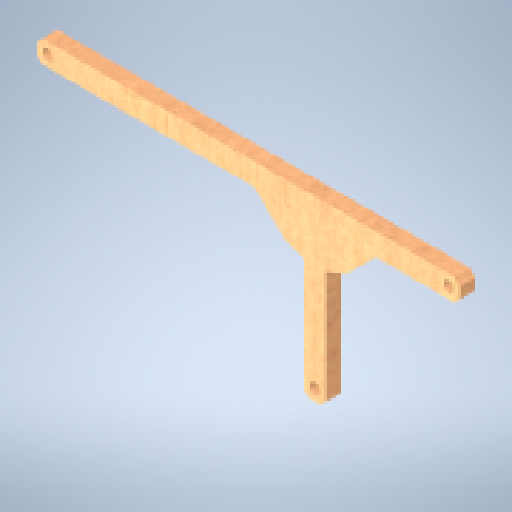
# Autodesk Inventor part: brazoT
Saved by Autodesk Inventor 2023.1 (Build 271208000, 208)
## iProperties
Created: 2022-10-30
Part Number: brazoT
Material: MDF Medium Density Fiberboard
Document SubType Name: Modeling
Designer: Daniel Peña
Density: 0.8 g/cm^3
Appearance: Cherry - Natural Low Gloss
Author: Daniel Peña
Autodesk Inventor part; units mm, degrees
ref_plane "YZ Plane" through (0, 0, 0) normal (1, 0, 0) x (0, 1, 0)
ref_plane "XZ Plane" through (0, 0, 0) normal (0, 1, 0) x (-1, 0, 0)
ref_plane "XY Plane" through (0, 0, 0) normal (0, 0, 1) x (1, 0, 0)
sketch "Sketch1" plane through (0, 0, 0) normal (0, 0, 1) x (1, 0, 0)
  circle A0 centre (-125, 70) radius 2.5 projected
  circle A1 centre (-185, 0.0856) radius 2.5 projected
  line L0 (-125, 70) -> (-305, 70) construction
  line L1 (-185, 0.0856) -> (-185, 70) construction
  line L2 (-310, 67.5) -> (-310, 72.5)
  line L3 (-307.5, 75) -> (-122.5, 75)
  line L4 (-120, 72.5) -> (-120, 67.5)
  line L5 (-180, 48.0357) -> (-180, -2.4144)
  line L6 (-182.5, -4.9144) -> (-187.5, -4.9144)
  line L7 (-190, -2.4144) -> (-190, 48.0357)
  line L8 (-122.5, 65) -> (-157.6881, 65)
  line L9 (-212.3119, 65) -> (-307.5, 65)
  line L10 (-120, 67.5) -> (-122.5, 65)
  line L11 (-120, 72.5) -> (-122.5, 75)
  line L12 (-180, -2.4144) -> (-182.5, -4.9144)
  line L13 (-187.5, -4.9144) -> (-190, -2.4144)
  line L14 (-307.5, 65) -> (-310, 67.5)
  line L15 (-307.5, 75) -> (-310, 72.5)
  line L16 (-170.7801, 51.9079) -> (-180, 48.0357)
  line L17 (-170.7801, 51.9079) -> (-157.6881, 65)
  line L18 (-199.2199, 51.9079) -> (-190, 48.0357)
  line L19 (-199.2199, 51.9079) -> (-212.3119, 65)
  point P0 (0, 0)
  point P1 (-120, 65)
  point P2 (-310, 75)
  point P3 (-310, 65)
  point P4 (-120, 75)
  point P5 (-180, -4.9144)
  point P6 (-190, -4.9144)
  point P7 (-161.5602, 55.7801)
  dimension "d0" = 180
  dimension "d1" = 60
  dimension "d2" = 5
  dimension "d3" = 5
  dimension "d4" = 5
  dimension "d5" = 5
  dimension "d6" = 5
  dimension "d7" = 2.5
  dimension "d8" = 2.5
  dimension "d9" = 2.5
  dimension "d10" = 2.5
  dimension "d11" = 2.5
  dimension "d12" = 2.5
  dimension "d13" = 2.5
  dimension "d14" = 2.5
  dimension "d15" = 2.5
  dimension "d16" = 2.5
  dimension "d17" = 2.5
  dimension "d18" = 2.5
  dimension "d19" = 20
  dimension "d20" = 10
  dimension "d21" = 10
  dimension "d22" = 10
  constraints: 40 end point, 14 point on line, 4 horizontal, 4 parallel, 3 perpendicular, 3 symmetric about line, 1 coincident, 1 collinear, 5 other
  measures "d0" distance of L0.start L0.end
  measures "d1" distance from line of L0.start L1
  measures "d2" distance between parallel lines of L3 L0
  measures "d3" distance from line of L0.start L4
  measures "d4" distance from line of L0.end L2
  measures "d5" distance between parallel lines of L5 L1
  measures "d6" distance from line of L1.start L6
  measures "d7" distance of L4.end point (-120, 65)
  measures "d8" distance of L8.start point (-120, 65)
  measures "d9" distance of L4.start point (-120, 75)
  measures "d10" distance of L3.end point (-120, 75)
  measures "d11" distance of L5.end point (-180, -4.914)
  measures "d12" distance of L6.start point (-180, -4.914)
  measures "d13" distance of L6.end point (-190, -4.914)
  measures "d14" distance of L7.start point (-190, -4.914)
  measures "d15" distance of L9.end point (-310, 65)
  measures "d16" distance of L2.start point (-310, 65)
  measures "d17" distance of L3.start point (-310, 75)
  measures "d18" distance of L2.end point (-310, 75)
  measures "d19" distance of L5.start point (-161.56, 55.78)
  measures "d20" distance of point (-157.688, 65) point (-161.56, 55.78)
  measures "d21" distance of L16.start point (-161.56, 55.78)
  measures "d22" distance of L8.end point (-161.56, 55.78)
extrude "Extrusion1" add sketch "Sketch1" along normal blind 7 contours A0 | A1 | L2 L15 L3 L11 L4 L10 L8 L17 L16 L5 L12 L6 L13 L7 L18 L19 L9 L14
sketch "Sketch2" plane through (0, 0, 7) normal (0, 0, 1) x (1, 0, 0)
  line L0 (-120, 67.5) -> (-120, 72.5) projected
  line L1 (-187.5, -4.9144) -> (-182.5, -4.9144) projected
  line L2 (-310, 72.5) -> (-310, 67.5) projected
  point P0 (0, 0)
  point P1 (-125, 70)
  point P2 (-305, 70)
  point P3 (-185, 0.0856)
  point P4 (-185, -4.9144)
  dimension "d25" = 5
  dimension "d26" = 5
  dimension "d27" = 5
  constraints: 1 midpoint
  measures "d25" distance from line of point (-125, 70) L0
  measures "d26" distance of point (-185, -4.914) point (-185, 0.086)
  measures "d27" distance from line of L2 point (-305, 70)
hole "Hole1" at (-125, 70, 7) at (-305, 70, 7) at (-185, 0.0856, 7) direction (0, 0, -1) diameter 5 end through all
sketch "Sketch3" plane through (0, 0, 7) normal (0, 0, 1) x (1, 0, 0)
  circle A0 centre (-185.0818, 61.5583) radius 12.5 construction
  point P0 (0, 0)
  dimension "d35" = 25
  constraints: 1 centre point
  measures "d35" diameter of A0
equation "\"d8\" = d7"
equation "\"d9\" = d7"
equation "\"d10\" = d9"
equation "\"d11\" = d7"
equation "\"d12\" = d11"
equation "\"d13\" = d7"
equation "\"d14\" = d13"
equation "\"d15\" = d7"
equation "\"d16\" = d15"
equation "\"d17\" = d7"
equation "\"d18\" = d17"
equation "\"d22\" = d21"
body "Solid1"
